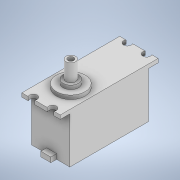
# Autodesk Inventor part: servo
Saved by Autodesk Inventor 2020 (Build 240168000, 168)
## iProperties
Created: 2019-06-06
Part Number: servo
Material: Generic
Document SubType Name: Modeling
Designer: Vivek Muskan
Density: 1 g/cm^3
Appearance: Default
Author: Vivek Muskan
Autodesk Inventor part; units mm, degrees
ref_plane "YZ Plane" through (0, 0, 0) normal (1, 0, 0) x (0, 1, 0)
ref_plane "XZ Plane" through (0, 0, 0) normal (0, 1, 0) x (-1, 0, 0)
sketch "Sketch1" plane through (0, 0, 0) normal (0, 1, 0) x (-1, 0, 0)
  line L0 (0, 0) -> (-20, 0)
  line L1 (-20, 0) -> (-20, -41)
  line L2 (-20, -41) -> (0, -41)
  line L3 (0, -41) -> (0, 0)
  dimension "d0" = 20
  dimension "d1" = 41
  constraints: 8 end point, 2 parallel, 1 horizontal, 1 perpendicular
  measures "d0" distance of L2.end L1.end
  measures "d1" distance of L1.end L0.end
extrude "Extrusion1" add sketch "Sketch1" along normal blind 24
sketch "Sketch2" plane through (0, 24, 0) normal (0, 1, 0) x (1, 0, 0)
  line L0 (0, 41) -> (0, 0) projected
  line L1 (0, 0) -> (0, -5)
  line L2 (0, -5) -> (20, -5)
  line L3 (20, -5) -> (20, 46)
  line L4 (20, 46) -> (0, 46)
  line L5 (0, 46) -> (0, -5)
  line L6 (0, -4) -> (5, -4)
  circle A0 centre (5, -4) radius 2
  line L7 (5, -4) -> (15, -4)
  circle A1 centre (15, -4) radius 2
  line L8 (0, 0) -> (0, 20.5)
  line L9 (0, 20.5) -> (20, 20.5)
  line L10 (20, 0) -> (20, 41) projected
  line L11 (0, 45) -> (5, 45)
  circle A2 centre (5, 45) radius 2
  circle A3 centre (15, 45) radius 2
  line L12 (0, 0) -> (20, 0) projected
  point P0 (3.2679, -5)
  point P1 (6.7321, -5)
  point P2 (13.2679, -5)
  point P3 (16.7321, -5)
  point P4 (16.7321, 46)
  point P5 (13.2679, 46)
  point P6 (6.7321, 46)
  point P7 (3.2679, 46)
  dimension "d4" = 5
  dimension "d5" = 20
  dimension "d6" = 51
  dimension "d7" = 5
  dimension "d8" = 4
  dimension "d9" = 10
  dimension "d10" = 4
  dimension "d11" = 20.5
  dimension "d29" = 4
  constraints: 20 end point, 4 centre point, 4 symmetric about line, 3 coincident, 2 horizontal, 2 midpoint, 2 parallel, 2 perpendicular, 1 point on line, 1 vertical, 2 other
  measures "d4" distance of L0.end L1.end
  measures "d5" distance of L4.end L3.end
  measures "d6" distance of L3.end L2.end
  measures "d7" distance of L6.start L6.end
  measures "d8" diameter of A0
  measures "d9" distance of L7.start L7.end
  measures "d10" diameter of A1
  measures "d11" distance of L0.end L8.end
  measures "d29" distance from line of L7.start L12
extrude "Extrusion2" add sketch "Sketch2" along normal blind 2 contours L5 L11 A2 L4 A3 L3 L9 L0 | L9 L3 L12 L0 | L5 L4 A2 L11 | L12 L3 L2 A1 L7 A0 L6 L1 | L6 A0 L2 L1 | L7 A1 L2 A0
sketch "Sketch3" plane through (0, 26, 0) normal (0, 1, 0) x (1, 0, 0)
  line L0 (0, 46) -> (0, -5) projected
  line L1 (0, -5) -> (0, 10)
  line L2 (0, 10) -> (10.5, 10)
  circle A0 centre (10.5, 10) radius 2.5
  circle A1 centre (10.5, 10) radius 4
  circle A2 centre (10.5, 10) radius 7.5
  circle A3 centre (10.5, 10) radius 1.5
  point P0 (0, 0)
  dimension "d14" = 15
  dimension "d15" = 10.5
  dimension "d16" = 5
  dimension "d17" = 8
  dimension "d18" = 15
  dimension "d19" = 3
  constraints: 4 centre point, 4 coincident, 4 end point, 1 perpendicular, 1 point on line
  measures "d14" distance of L0.end L1.end
  measures "d15" distance of L1.end L2.end
  measures "d16" diameter of A0
  measures "d17" diameter of A1
  measures "d18" diameter of A2
  measures "d19" diameter of A3
extrude "Extrusion3" add sketch "Sketch3" along normal blind 13 contours A0
extrude "Extrusion4" add sketch "Sketch3" along normal blind 4 contours A1
extrude "Extrusion5" add sketch "Sketch3" along normal blind 2 contours A2
sketch "Sketch4" plane through (0, 0, 0) normal (0, 0, 1) x (1, 0, 0)
  line L0 (20, 0) -> (0, 0) projected
  line L1 (7.8843, 0) -> (13.1114, 0)
  line L2 (13.1114, 0) -> (13.1114, 2.57)
  line L3 (13.1114, 2.57) -> (7.8843, 2.57)
  line L4 (7.8843, 2.57) -> (7.8843, 0)
  constraints: 8 end point, 2 parallel, 1 horizontal, 1 perpendicular, 1 point on line
extrude "Extrusion6" add sketch "Sketch4" along normal blind 3
ref_plane "Work Plane1" through (0, 56, 0) normal (0, 1, 0) x (1, 0, 0)
sketch "Sketch5" plane through (0, 56, 0) normal (0, 1, 0) x (1, 0, 0)
  circle A0 centre (10.5, 10) radius 7.5 projected
  line L0 (0, 46) -> (0, -5) projected
  line L1 (0, -5) -> (3.2679, -5) projected
  arc A1 (6.7321, -5) -> (3.2679, -5) centre (5, -4) ccw projected
  line L2 (6.7321, -5) -> (13.2679, -5) projected
  arc A2 (16.7321, -5) -> (13.2679, -5) centre (15, -4) ccw projected
  line L3 (16.7321, -5) -> (20, -5) projected
  line L4 (20, -5) -> (20, 46) projected
  line L5 (20, 46) -> (16.7321, 46) projected
  arc A3 (13.2679, 46) -> (16.7321, 46) centre (15, 45) ccw projected
  line L6 (13.2679, 46) -> (6.7321, 46) projected
  arc A4 (3.2679, 46) -> (6.7321, 46) centre (5, 45) ccw projected
  line L7 (3.2679, 46) -> (0, 46) projected
  circle A5 centre (10.5, 10) radius 2.5 projected
  circle A6 centre (10.5, 10) radius 4 projected
  circle A7 centre (10.5, 10) radius 1.5 projected
  point P0 (0, 0)
body "Solid1"
